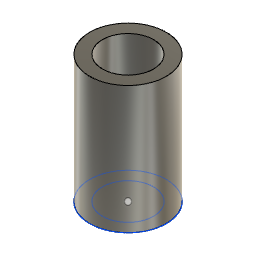
10mm height (Autodesk Fusion 360 design; units mm, degrees)
Autodesk Fusion 360 part; units mm, degrees
sketch "Sketch1" plane through (0, 0, 0) normal (0, 0, 1) x (1, 0, 0)
  circle A0 centre (0, 0) radius 3
  circle A1 centre (0, 0) radius 2
  dimension "d4" = 6
  dimension "d8" = 4
  constraint concentric A0 A1
  measures "d4" diameter of A0
  measures "d8" diameter of A1
extrude "Extrude1" add sketch "Sketch1" along normal blind 10 contours A0 | A1
extrude "Extrude2" cut sketch "Sketch1" along normal blind 100 contours A1
equation "inner_radius = 2 mm"
equation "outer_radius = 3 mm"
equation "height = 10 mm"
equation "d4 = outer_radius * 2"
equation "extra = 100 mm"
equation "d6 = height"
equation "d8 = inner_radius * 2"
equation "d9 = extra"
